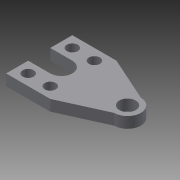
# Autodesk Inventor part: Model
Saved by Autodesk Inventor 2015 SP1 (Build 190203100, 203)
## iProperties
Created: 2015-11-06
Part Number: Model
Material: Типовые
Document SubType Name: Modeling
Designer: 1
Density: 1 g/cm^3
Appearance: По умолчанию
Author: 1
Autodesk Inventor part; units mm, degrees
ref_plane "YZ Plane" through (0, 0, 0) normal (1, 0, 0) x (0, 1, 0)
ref_plane "XZ Plane" through (0, 0, 0) normal (0, 1, 0) x (-1, 0, 0)
ref_plane "XY Plane" through (0, 0, 0) normal (0, 0, 1) x (1, 0, 0)
sketch "Эскиз1" plane through (0, 0, 0) normal (0, 0, 1) x (1, 0, 0)
  line L0 (-18.1191, -2.1753) -> (21.8809, -2.1753)
  line L1 (-18.1191, -2.1753) -> (-18.1191, 17.8247)
  line L2 (-18.1191, 17.8247) -> (1.8809, 17.8247)
  line L3 (-18.1191, 57.8247) -> (-18.1191, 37.8247)
  line L4 (-18.1191, 37.8247) -> (1.8809, 37.8247)
  line L5 (-18.1191, 57.8247) -> (21.8809, 57.8247)
  arc A0 (1.8809, 17.8247) -> (1.8809, 37.8247) centre (1.8809, 27.8247) ccw
  circle A1 centre (61.8809, 27.8247) radius 7.5
  line L6 (21.8809, 57.8247) -> (61.8809, 39.8247)
  line L7 (21.8809, -2.1753) -> (61.8809, 15.8247)
  arc A2 (61.8809, 15.8247) -> (61.8809, 39.8247) centre (61.8809, 27.8247) ccw
  circle A3 centre (-8.1191, 47.8247) radius 5
  circle A4 centre (-8.1191, 7.8247) radius 5
  circle A5 centre (11.8809, 47.8247) radius 5
  circle A6 centre (11.8809, 7.8247) radius 5
  point P0 (0, 0)
  dimension "j" = 40
  dimension "p" = 20
  dimension "g1" = 20
  dimension "d" = 60
  dimension "p1" = 20
  dimension "R1" = 15
  dimension "t" = 12
  dimension "r" = 10
  dimension "u" = 20
  dimension "a" = 80
  dimension "f1" = 10
  constraints: 16 end point, 7 centre point, 4 point on circle, 3 horizontal, 2 tangent, 1 perpendicular, 1 vertical
  measures "j" distance of L0.start L0.end
  measures "p" distance of L0.start L1.end
  measures "g1" distance of L1.end L2.end
  measures "d" distance of L0.start L3.start
  measures "p1" distance of L3.start L3.end
  measures "R1" diameter of A1
  measures "t" distance of A1.centre L6.end
  measures "r" diameter of A5
  measures "u" distance of A5.centre A3.centre
  measures "a" horizontal distance of A1.centre L1.end
  measures "f1" distance from line of L5 A3.centre
sketch "Эскиз2" plane through (0, 0, 0) normal (0, 0, 1) x (1, 0, 0)
  point P0 (0, 0)
sketch "Эскиз3" plane through (0, 0, 0) normal (0, 0, 1) x (1, 0, 0)
  point P0 (0, 0)
extrude "Выдавливание1" add sketch "Эскиз1" along normal blind 10
